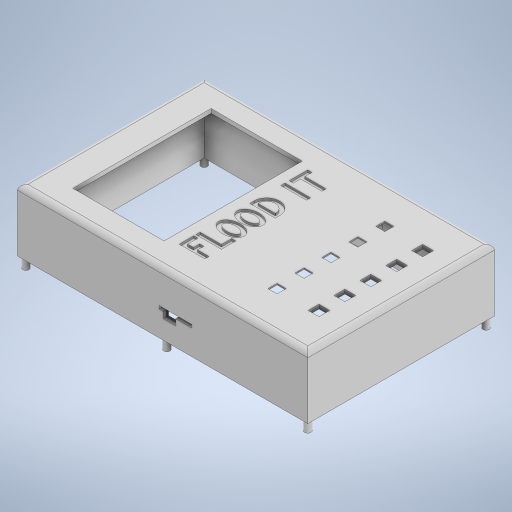
# Autodesk Inventor part: CaseTop3.0
Saved by Autodesk Inventor 2023 (Build 270158000, 158)
## iProperties
Created: 2022-11-29
Part Number: CaseTop3.0
Material: Generic
Document SubType Name: Modeling
Designer: spfow
Density: 1 g/cm^3
Appearance: Default
Author: spfow
Autodesk Inventor part; units mm, degrees
note: some values were not read from the file. Chosen so that the rebuilt part matches the saved one: offset side.
ref_plane "YZ Plane" through (0, 0, 0) normal (1, 0, 0) x (0, 1, 0)
ref_plane "XZ Plane" through (0, 0, 0) normal (0, 1, 0) x (-1, 0, 0)
ref_plane "XY Plane" through (0, 0, 0) normal (0, 0, 1) x (1, 0, 0)
sketch "Sketch1" plane through (0, 0, 0) normal (0, 1, 0) x (-1, 0, 0)
  line L0 (0, 0) -> (177.8, 0)
  line L1 (177.8, 0) -> (177.8, -114.3)
  line L2 (177.8, -114.3) -> (0, -114.3)
  line L3 (0, -114.3) -> (0, 0)
  dimension "d0" = 177.8
  dimension "d1" = 114.3
  constraints: 8 end point, 2 parallel, 1 horizontal, 1 perpendicular
  measures "d0" distance of L1.end L2.end
  measures "d1" distance of L0.end L1.end
extrude "Extrusion1" add sketch "Sketch1" along normal blind 38.1
sketch "Sketch2" plane through (0, 0, 0) normal (0, -1, 0) x (1, 0, 0)
  line L0 (-177.8, -114.3) -> (-177.8, 0) projected
  line L1 (0, 0) -> (-177.8, 0)
  line L2 (-177.8, 0) -> (-177.8, -114.3)
  line L3 (-177.8, -114.3) -> (0, -114.3)
  line L4 (0, -114.3) -> (0, 0)
  line L5 (-5.08, -5.08) -> (-172.72, -5.08)
  line L6 (-172.72, -5.08) -> (-172.72, -109.22)
  line L7 (-172.72, -109.22) -> (-5.08, -109.22)
  line L8 (-5.08, -109.22) -> (-5.08, -5.08)
  dimension "d4" = 5.08
  constraints: 16 end point, 4 parallel, 2 perpendicular, 1 horizontal, 3 other
  measures "d4" distance between parallel lines of L4 L8
extrude "Extrusion2" cut sketch "Sketch2" against normal blind 35.56 contours L8 L7 L6 L5
fillet "Fillet1" radius 3.175 4 edges at (-177.8, 38.1, -57.15) (-88.9, 38.1, 0) (-88.9, 38.1, -114.3) (0, 38.1, -57.15)
sketch "Sketch3" plane through (0, 38.1, 0) normal (0, 1, 0) x (1, 0, 0)
  line L0 (-177.8, 114.3) -> (-171.45, 114.3)
  line L1 (-171.45, 114.3) -> (-171.45, 0)
  line L2 (-171.45, 0) -> (-177.8, 0)
  line L3 (-177.8, 0) -> (-177.8, 114.3)
  line L4 (0, 114.3) -> (-177.8, 114.3) projected
  line L5 (-177.8, 114.3) -> (0, 114.3)
  line L6 (0, 114.3) -> (0, 107.95)
  line L7 (0, 107.95) -> (-177.8, 107.95)
  line L8 (-177.8, 107.95) -> (-177.8, 114.3)
  line L9 (-158.75, 99.5045) -> (-102.87, 99.5045)
  line L10 (-102.87, 99.5045) -> (-102.87, 14.7955)
  line L11 (-102.87, 14.7955) -> (-158.75, 14.7955)
  line L12 (-158.75, 14.7955) -> (-158.75, 99.5045)
  point P0 (0, 0)
  dimension "d8" = 6.35
  dimension "d9" = 6.35
  dimension "d10" = 55.88
  dimension "d11" = 84.709
  dimension "d12" = 14.7955
  dimension "d13" = 19.05
  constraints: 24 end point, 6 parallel, 3 horizontal, 3 perpendicular
  measures "d8" distance of L1.end L2.end
  measures "d9" distance of L5.end L6.end
  measures "d10" distance of L9.start L9.end
  measures "d11" distance of L9.end L10.end
  measures "d12" distance between parallel lines of L4 L9
  measures "d13" distance between parallel lines of L3 L12
extrude "Extrusion3" cut sketch "Sketch3" against normal blind 35.56 contours L9 L10 L11 L12
sketch "Sketch4" plane through (0, 38.1, 0) normal (0, 1, 0) x (1, 0, 0)
  line L0 (-96.52, 17.78) -> (-81.2088, 17.78)
  line L1 (-93.98, 20.32) -> (-93.98, 26.67)
  line L2 (-93.98, 26.67) -> (-96.52, 26.67)
  line L3 (-96.52, 26.67) -> (-96.52, 17.78)
  line L4 (-96.52, 17.78) -> (-80.899, 17.78)
  line L5 (-80.899, 17.78) -> (-80.899, 20.32)
  line L6 (-96.52, 23.1535) -> (-96.52, 17.78)
  line L7 (-87.884, 20.32) -> (-87.884, 24.13)
  line L8 (-87.884, 24.13) -> (-90.424, 24.13)
  line L9 (-90.424, 24.13) -> (-90.424, 20.32)
  line L10 (-80.899, 20.32) -> (-87.884, 20.32)
  line L11 (-90.424, 20.32) -> (-93.98, 20.32)
  line L12 (-102.87, 99.5045) -> (-102.87, 14.7955) projected
  line L13 (-177.8, 0) -> (0, 0) projected
  line L14 (-96.52, 27.94) -> (-80.899, 27.94)
  line L15 (-80.899, 27.94) -> (-80.899, 30.7699)
  line L16 (-83.439, 30.48) -> (-96.52, 30.48)
  line L17 (-96.52, 30.48) -> (-96.52, 27.94)
  line L18 (-83.0828, 27.94) -> (-80.899, 27.94)
  line L19 (-80.899, 27.94) -> (-80.899, 36.83)
  line L20 (-80.899, 36.83) -> (-83.439, 36.83)
  line L21 (-83.439, 36.83) -> (-83.439, 30.48)
  ellipse E0 centre (-88.7095, 41.91) end of major axis (-96.52, 41.91) minor radius 5.334
  ellipse E1 centre (-88.7095, 53.34) end of major axis (-96.52, 53.34) minor radius 5.334
  line L22 (-96.52, 60.96) -> (-80.899, 60.96)
  line L23 (-80.899, 60.96) -> (-80.899, 63.754)
  line L24 (-96.52, 63.754) -> (-96.52, 60.96)
  ellipse E2 centre (-88.7095, 63.754) end of major axis (-96.52, 63.754) minor radius 7.62 (-80.899, 63.754) -> (-96.52, 63.754) ccw
  line L25 (-93.98, 63.754) -> (-93.98, 63.5)
  line L26 (-93.98, 63.5) -> (-83.439, 63.5)
  line L27 (-83.439, 63.5) -> (-83.439, 63.754)
  line L28 (-96.52, 82.55) -> (-80.899, 82.55)
  line L29 (-80.899, 82.55) -> (-80.899, 80.01)
  line L30 (-80.899, 80.01) -> (-96.52, 80.01)
  line L31 (-96.52, 80.01) -> (-96.52, 82.55)
  line L32 (-93.98, 89.535) -> (-80.899, 89.535)
  line L33 (-80.899, 89.535) -> (-80.899, 92.075)
  line L34 (-80.899, 92.075) -> (-93.98, 92.075)
  line L35 (-96.52, 94.8241) -> (-96.52, 91.9305)
  line L36 (-96.52, 85.09) -> (-93.98, 85.09)
  line L37 (-93.98, 96.52) -> (-96.52, 96.52)
  line L38 (-96.52, 96.52) -> (-96.52, 85.09)
  line L39 (-93.98, 85.09) -> (-93.98, 89.535)
  line L40 (-93.98, 92.075) -> (-93.98, 96.52)
  spline S0 degree 5 poles (-93.98, 41.91) (-93.9809, 41.6813) (-93.9169, 41.4527) (-93.811, 41.2473) (-93.4267, 40.6846) (-92.8861, 40.2564) (-92.5045, 40.0177) (-91.5531, 39.5478) (-90.5271, 39.2718) (-89.9251, 39.1679) (-88.7095, 39.0641) (-87.4939, 39.1679) (-86.8919, 39.2718) (-85.866, 39.5478) (-84.9145, 40.0176) (-84.5332, 40.2563) (-83.9921, 40.6845) (-83.6083, 41.2473) (-83.5012, 41.4526) (-83.3764, 41.91) (-83.5012, 42.3674) (-83.6083, 42.5727) (-83.9921, 43.1355) (-84.5332, 43.5637) (-84.9145, 43.8024) (-85.866, 44.2722) (-86.8919, 44.5482) (-87.4939, 44.6521) (-88.7095, 44.7559) (-89.9251, 44.6521) (-90.5271, 44.5482) (-91.5531, 44.2722) (-92.5045, 43.8023) (-92.8861, 43.5636) (-93.4267, 43.1354) (-93.811, 42.5727) (-93.9169, 42.3673) (-93.9809, 42.1387) (-93.98, 41.91) knots 0 0 0 0 0 0 0.044471 0.044471 0.044471 0.131758 0.131758 0.131758 0.25 0.25 0.25 0.36824 0.36824 0.36824 0.455522 0.455522 0.455522 0.5 0.5 0.5 0.544478 0.544478 0.544478 0.63176 0.63176 0.63176 0.75 0.75 0.75 0.868242 0.868242 0.868242 0.955529 0.955529 0.955529 1 1 1 1 1 1
  spline S1 degree 5 poles (-93.98, 53.34) (-93.9809, 53.1113) (-93.9169, 52.8827) (-93.811, 52.6773) (-93.4267, 52.1146) (-92.8861, 51.6864) (-92.5045, 51.4477) (-91.5531, 50.9778) (-90.5271, 50.7018) (-89.9251, 50.5979) (-88.7095, 50.4941) (-87.4939, 50.5979) (-86.8919, 50.7018) (-85.866, 50.9778) (-84.9145, 51.4476) (-84.5332, 51.6863) (-83.9921, 52.1145) (-83.6083, 52.6773) (-83.5012, 52.8826) (-83.3764, 53.34) (-83.5012, 53.7974) (-83.6083, 54.0027) (-83.9921, 54.5655) (-84.5332, 54.9937) (-84.9145, 55.2324) (-85.866, 55.7022) (-86.8919, 55.9782) (-87.4939, 56.0821) (-88.7095, 56.1859) (-89.9251, 56.0821) (-90.5271, 55.9782) (-91.5531, 55.7022) (-92.5045, 55.2323) (-92.8861, 54.9936) (-93.4267, 54.5654) (-93.811, 54.0027) (-93.9169, 53.7973) (-93.9809, 53.5687) (-93.98, 53.34) knots 0 0 0 0 0 0 0.044471 0.044471 0.044471 0.131758 0.131758 0.131758 0.25 0.25 0.25 0.36824 0.36824 0.36824 0.455522 0.455522 0.455522 0.5 0.5 0.5 0.544478 0.544478 0.544478 0.63176 0.63176 0.63176 0.75 0.75 0.75 0.868242 0.868242 0.868242 0.955529 0.955529 0.955529 1 1 1 1 1 1
  spline S2 degree 5 poles (-83.439, 63.754) (-83.4391, 64.309) (-83.5178, 64.8639) (-83.675, 65.404) (-84.3507, 66.8995) (-85.581, 68.0474) (-86.5678, 68.5716) (-88.7095, 69.0964) (-90.8512, 68.5716) (-91.838, 68.0474) (-93.0683, 66.8995) (-93.744, 65.404) (-93.9012, 64.8639) (-93.9799, 64.309) (-93.98, 63.754) knots 0 0 0 0 0 0 0.170659 0.170659 0.170659 0.5 0.5 0.5 0.829341 0.829341 0.829341 1 1 1 1 1 1
  point P0 (-96.52, 93.3773)
  point P1 (-88.9, 0)
  point P2 (-95.25, 85.09)
  dimension "d32" = 5.334
  dimension "d33" = 7.8105
  dimension "d36" = 7.8105
  dimension "d37" = 5.334
  dimension "d42" = 7.62
  dimension "d43" = 2.54
  dimension "d16" = 2.54
  dimension "d17" = 3.556
  dimension "d18" = 2.54
  dimension "d19" = 6.985
  dimension "d20" = 8.89
  dimension "d21" = 6.35
  dimension "d22" = 3.81
  dimension "d23" = 3.81
  dimension "d24" = 6.35
  dimension "d25" = 17.78
  dimension "d26" = 2.54
  dimension "d27" = 2.54
  dimension "d28" = 6.35
  dimension "d29" = 15.621
  dimension "d30" = 6.35
  dimension "d31" = 27.94
  dimension "d34" = 14.1605
  dimension "d35" = 41.91
  dimension "d38" = 14.1605
  dimension "d39" = 53.34
  dimension "d40" = 2.54
  dimension "d41" = 2.54
  dimension "d44" = 6.35
  dimension "d45" = 15.621
  dimension "d46" = 60.96
  dimension "d47" = 2.794
  dimension "d48" = 63.754
  dimension "d49" = 14.1605
  dimension "d50" = 2.54
  dimension "d51" = 15.621
  dimension "d52" = 4.445
  dimension "d53" = 4.445
  dimension "d54" = 2.54
  dimension "d55" = 2.54
  dimension "d56" = 6.35
  dimension "d57" = 80.01
  dimension "d58" = 2.54
  dimension "d59" = 13.081
  dimension "d62" = 2.9845
  dimension "d63" = 2.9845
  constraints: 78 end point, 20 parallel, 10 perpendicular, 8 horizontal, 5 point on line, 3 midpoint, 13 other
  measures "d16" distance of L1.end L2.end
  measures "d17" distance of L9.end L1.start
  measures "d18" distance of L7.end L8.end
  measures "d19" distance of L5.end L7.start
  measures "d20" distance of L2.end L0.start
  measures "d21" distance of L1.start L1.end
  measures "d22" distance of L8.end L9.end
  measures "d23" distance of L7.start L7.end
  measures "d24" distance between parallel lines of L12 L3
  measures "d25" distance between parallel lines of L13 L0
  measures "d26" distance of L16.end L14.start
  measures "d27" distance of L19.end L20.end
  measures "d28" distance of L20.end L16.start
  measures "d29" distance of L14.start L14.end
  measures "d30" distance between parallel lines of L12 L17
  measures "d31" distance between parallel lines of L13 L14
  measures "d34" distance from line of L12 point (-88.71, 41.91)
  measures "d35" distance from line of L13 point (-88.71, 41.91)
  measures "d38" distance from line of L12 point (-88.71, 53.34)
  measures "d39" distance from line of L13 point (-88.71, 53.34)
  measures "d44" distance between parallel lines of L12 L24
  measures "d45" distance of L22.start L22.end
  measures "d46" distance between parallel lines of L13 L22
  measures "d47" distance of L24.start L22.start
  measures "d48" distance from line of L13 point (-88.71, 63.754)
  measures "d49" distance from line of L12 point (-88.71, 63.754)
  measures "d50" distance of L30.end L28.start
  measures "d51" distance of L29.end L30.end
  measures "d52" distance of L36.end L32.start
  measures "d53" distance of L34.end L37.start
  measures "d54" distance between parallel lines of L32 L34
  measures "d55" distance between parallel lines of L40 L38
  measures "d56" distance from line of L12 point (-96.52, 93.377)
  measures "d57" distance from line of point (-88.9, 0) L30
  measures "d58" distance from line of L28 point (-95.25, 85.09)
  measures "d59" distance of L32.start L32.end
  measures "d62" distance from line of L12.start L37
  measures "d63" distance from line of L12.end L0
extrude "Extrusion4" cut sketch "Sketch4" against normal blind 1.27
sketch "Sketch5" plane through (0, 38.1, 0) normal (0, 1, 0) x (1, 0, 0)
  line L0 (-45.72, 21.3678) -> (-40.1955, 21.3678)
  line L1 (-40.1955, 21.3678) -> (-40.1955, 26.8923)
  line L2 (-40.1955, 26.8923) -> (-45.72, 26.8923)
  line L3 (-45.72, 26.8923) -> (-45.72, 21.3678)
  line L4 (-45.72, 37.8778) -> (-40.1955, 37.8778)
  line L5 (-40.1955, 37.8778) -> (-40.1955, 43.4023)
  line L6 (-40.1955, 43.4023) -> (-45.72, 43.4023)
  line L7 (-45.72, 43.4023) -> (-45.72, 37.8778)
  line L8 (-45.72, 54.3877) -> (-40.1955, 54.3877)
  line L9 (-40.1955, 54.3877) -> (-40.1955, 59.9123)
  line L10 (-40.1955, 59.9123) -> (-45.72, 59.9123)
  line L11 (-45.72, 59.9123) -> (-45.72, 54.3877)
  line L12 (-45.72, 70.8978) -> (-40.1955, 70.8978)
  line L13 (-40.1955, 70.8978) -> (-40.1955, 76.4222)
  line L14 (-40.1955, 76.4222) -> (-45.72, 76.4222)
  line L15 (-45.72, 76.4222) -> (-45.72, 70.8978)
  line L16 (-45.72, 87.4077) -> (-40.1955, 87.4077)
  line L17 (-40.1955, 87.4077) -> (-40.1955, 92.9322)
  line L18 (-40.1955, 92.9322) -> (-45.72, 92.9322)
  line L19 (-45.72, 92.9322) -> (-45.72, 87.4077)
  line L20 (0, 114.3) -> (-177.8, 114.3) projected
  line L21 (-177.8, 0) -> (0, 0) projected
  line L22 (-102.87, 99.5045) -> (-102.87, 14.7955) projected
  point P0 (-45.72, 73.66)
  dimension "d64" = 5.5245
  dimension "d65" = 5.5245
  dimension "d66" = 5.5245
  dimension "d67" = 5.5245
  dimension "d68" = 5.5245
  dimension "d69" = 5.5245
  dimension "d70" = 16.51
  dimension "d71" = 16.51
  dimension "d72" = 16.51
  dimension "d73" = 16.51
  dimension "d74" = 21.3678
  dimension "d76" = 57.15
  dimension "d224" = 21.3678
  constraints: 40 end point, 10 parallel, 8 point on line, 5 horizontal, 5 perpendicular, 1 midpoint
  measures "d64" distance of L2.end L0.start
  measures "d65" distance of L6.end L4.start
  measures "d66" distance of L10.end L8.start
  measures "d67" distance of L14.end L12.start
  measures "d68" distance of L18.end L16.start
  measures "d69" distance of L17.end L18.end
  measures "d70" distance of L5.end L1.end
  measures "d71" distance of L9.end L5.end
  measures "d72" distance of L13.end L9.end
  measures "d73" distance of L17.end L13.end
  measures "d74" distance between parallel lines of L20 L18
  measures "d76" distance from line of point (-45.72, 73.66) L22
  measures "d224" distance between parallel lines of L21 L0
extrude "Extrusion5" cut sketch "Sketch5" against normal blind 25.4
sketch "Sketch6" plane through (0, 35.56, 0) normal (0, -1, 0) x (1, 0, 0)
  line L0 (-45.72, -87.4077) -> (-45.72, -92.9322) projected
  line L1 (-45.72, -92.9322) -> (-40.1955, -92.9322)
  line L2 (-40.1955, -92.9322) -> (-40.1955, -87.4077)
  line L3 (-40.1955, -87.4077) -> (-45.72, -87.4077)
  line L4 (-45.72, -87.4077) -> (-45.72, -92.9322)
  line L5 (-45.72, -76.4222) -> (-40.1955, -76.4222) projected
  line L6 (-45.72, -70.8978) -> (-40.1955, -70.8978) projected
  line L7 (-45.72, -76.4222) -> (-40.1955, -76.4222)
  line L8 (-40.1955, -76.4222) -> (-40.1955, -70.8978)
  line L9 (-40.1955, -70.8978) -> (-45.72, -70.8978)
  line L10 (-45.72, -70.8978) -> (-45.72, -76.4222)
  line L11 (-45.72, -54.3877) -> (-45.72, -59.9123) projected
  line L12 (-45.72, -54.3877) -> (-40.1955, -54.3877) projected
  line L13 (-45.72, -59.9123) -> (-40.1955, -59.9123)
  line L14 (-40.1955, -59.9123) -> (-40.1955, -54.3877)
  line L15 (-40.1955, -54.3877) -> (-45.72, -54.3877)
  line L16 (-45.72, -54.3877) -> (-45.72, -59.9123)
  line L17 (-45.72, -37.8778) -> (-45.72, -43.4023) projected
  line L18 (-40.1955, -37.8778) -> (-45.72, -37.8778) projected
  line L19 (-45.72, -43.4023) -> (-40.1955, -43.4023)
  line L20 (-40.1955, -43.4023) -> (-40.1955, -37.8778)
  line L21 (-40.1955, -37.8778) -> (-45.72, -37.8778)
  line L22 (-45.72, -37.8778) -> (-45.72, -43.4023)
  line L23 (-45.72, -21.3678) -> (-45.72, -26.8923) projected
  line L24 (-45.72, -26.8923) -> (-40.1955, -26.8923)
  line L25 (-40.1955, -26.8923) -> (-40.1955, -21.3678)
  line L26 (-40.1955, -21.3678) -> (-45.72, -21.3678)
  line L27 (-45.72, -21.3678) -> (-45.72, -26.8923)
  line L28 (-46.736, -86.3917) -> (-39.1795, -86.3917)
  line L29 (-39.1795, -86.3917) -> (-39.1795, -93.9483)
  line L30 (-39.1795, -93.9483) -> (-46.736, -93.9483)
  line L31 (-46.736, -93.9483) -> (-46.736, -86.3917)
  line L32 (-46.736, -77.4383) -> (-39.1795, -77.4383)
  line L33 (-39.1795, -77.4383) -> (-39.1795, -69.8817)
  line L34 (-39.1795, -69.8817) -> (-46.736, -69.8817)
  line L35 (-46.736, -69.8817) -> (-46.736, -77.4383)
  line L36 (-39.1795, -60.9282) -> (-46.736, -60.9282)
  line L37 (-46.736, -60.9282) -> (-46.736, -53.3718)
  line L38 (-46.736, -53.3718) -> (-39.1795, -53.3718)
  line L39 (-39.1795, -53.3718) -> (-39.1795, -60.9282)
  line L40 (-39.1795, -44.4182) -> (-46.736, -44.4182)
  line L41 (-46.736, -44.4182) -> (-46.736, -36.8618)
  line L42 (-46.736, -36.8618) -> (-39.1795, -36.8618)
  line L43 (-39.1795, -36.8618) -> (-39.1795, -44.4182)
  line L44 (-39.1795, -27.9082) -> (-46.736, -27.9082)
  line L45 (-46.736, -27.9082) -> (-46.736, -20.3518)
  line L46 (-46.736, -20.3518) -> (-39.1795, -20.3518)
  line L47 (-39.1795, -20.3518) -> (-39.1795, -27.9082)
  line L48 (-49.1173, -100.3999) -> (-36.7983, -100.3999)
  line L49 (-36.7983, -100.3999) -> (-36.7983, -15.9449)
  line L50 (-36.7983, -15.9449) -> (-49.1173, -15.9449)
  line L51 (-49.1173, -15.9449) -> (-49.1173, -100.3999)
  line L52 (-21.844, -22.098) -> (-15.24, -22.098)
  line L53 (-15.24, -22.098) -> (-15.24, -28.702)
  line L54 (-15.24, -28.702) -> (-21.844, -28.702)
  line L55 (-21.844, -28.702) -> (-21.844, -22.098)
  line L56 (-21.844, -44.577) -> (-21.844, -37.973)
  line L57 (-15.24, -37.973) -> (-15.24, -44.577)
  line L58 (-15.24, -44.577) -> (-21.844, -44.577)
  line L59 (-21.844, -37.973) -> (-15.24, -37.973)
  line L60 (-21.844, -60.452) -> (-21.844, -53.848)
  line L61 (-15.24, -53.848) -> (-15.24, -60.452)
  line L62 (-15.24, -60.452) -> (-21.844, -60.452)
  line L63 (-21.844, -53.848) -> (-15.24, -53.848)
  line L64 (-21.844, -76.327) -> (-21.844, -69.723)
  line L65 (-15.24, -69.723) -> (-15.24, -76.327)
  line L66 (-15.24, -76.327) -> (-21.844, -76.327)
  line L67 (-21.844, -69.723) -> (-15.24, -69.723)
  line L68 (-21.844, -92.202) -> (-21.844, -85.598)
  line L69 (-15.24, -85.598) -> (-15.24, -92.202)
  line L70 (-15.24, -92.202) -> (-21.844, -92.202)
  line L71 (-21.844, -85.598) -> (-15.24, -85.598)
  line L72 (-172.72, -5.08) -> (-5.08, -5.08) projected
  line L73 (-5.08, -109.22) -> (-172.72, -109.22) projected
  line L74 (-5.08, -5.08) -> (-5.08, -109.22) projected
  point P0 (0, 0)
  point P1 (-42.9578, -93.9483)
  point P2 (-42.9578, -100.3999)
  point P3 (-42.9578, -15.9449)
  point P4 (-42.9578, -20.3518)
  dimension "d189" = 1.016
  dimension "d190" = 1.016
  dimension "d191" = 1.016
  dimension "d192" = 1.016
  dimension "d193" = 1.016
  dimension "d194" = 12.319
  dimension "d195" = 2.3813
  dimension "d197" = 84.455
  dimension "d198" = 6.4516
  dimension "d199" = 4.4069
  dimension "d248" = 6.604
  dimension "d249" = 6.604
  dimension "d252" = 15.875
  dimension "d257" = 17.018
  dimension "d258" = 17.018
  dimension "d259" = 10.16
  constraints: 128 end point, 24 parallel, 12 perpendicular, 7 horizontal, 4 midpoint, 1 collinear, 1 vertical, 46 other
  measures "d189" distance between parallel lines of L3 L28
  measures "d190" distance between parallel lines of L10 L35
  measures "d191" distance between parallel lines of L13 L36
  measures "d192" distance between parallel lines of L19 L40
  measures "d193" distance between parallel lines of L24 L44
  measures "d194" distance of L49.end L50.end
  measures "d195" distance between parallel lines of L31 L51
  measures "d197" distance of L50.end L48.start
  measures "d198" distance of point (-42.958, -93.948) point (-42.958, -100.4)
  measures "d199" distance of point (-42.958, -15.945) point (-42.958, -20.352)
  measures "d248" distance of L53.end L54.end
  measures "d249" distance of L52.end L53.end
  measures "d252" distance of L54.end L56.start
  measures "d257" distance between parallel lines of L72 L52
  measures "d258" distance between parallel lines of L73 L70
  measures "d259" distance between parallel lines of L74 L53
extrude "Extrusion9" cut sketch "Sketch6" against normal blind 1.7463 contours L28 L29 L30 L31 | L35 L34 L33 L32 | L36 L37 L38 L39 | L40 L41 L42 L43 | L44 L45 L46 L47
sketch "Sketch8" plane through (0, 35.56, 0) normal (0, -1, 0) x (1, 0, 0)
  line L0 (-102.87, -14.7955) -> (-102.87, -99.5045) projected
  line L1 (-102.87, -14.7955) -> (-160.9725, -14.7955)
  line L2 (-160.9725, -14.7955) -> (-160.9725, -8.4455)
  line L3 (-160.9725, -8.4455) -> (-102.87, -8.4455)
  line L4 (-102.87, -8.4455) -> (-102.87, -14.7955)
  line L5 (-158.75, -99.5045) -> (-102.87, -99.5045) projected
  line L6 (-102.87, -99.5045) -> (-160.9725, -99.5045)
  line L7 (-160.9725, -99.5045) -> (-160.9725, -106.4895)
  line L8 (-160.9725, -106.4895) -> (-102.87, -106.4895)
  line L9 (-102.87, -106.4895) -> (-102.87, -99.5045)
  line L10 (-102.87, -8.4455) -> (-96.52, -8.4455)
  line L11 (-96.52, -8.4455) -> (-96.52, -14.7955)
  line L12 (-96.52, -14.7955) -> (-102.87, -14.7955)
  line L13 (-102.87, -14.7955) -> (-102.87, -8.4455)
  line L14 (-102.87, -99.5045) -> (-96.52, -99.5045)
  line L15 (-96.52, -99.5045) -> (-96.52, -106.4895)
  line L16 (-96.52, -106.4895) -> (-102.87, -106.4895)
  line L17 (-102.87, -106.4895) -> (-102.87, -99.5045)
  line L18 (-160.9725, -99.5045) -> (-167.3225, -99.5045)
  line L19 (-167.3225, -99.5045) -> (-167.3225, -106.4895)
  line L20 (-167.3225, -106.4895) -> (-160.9725, -106.4895)
  line L21 (-160.9725, -106.4895) -> (-160.9725, -99.5045)
  line L22 (-160.9725, -8.4455) -> (-167.3225, -8.4455)
  line L23 (-167.3225, -8.4455) -> (-167.3225, -12.827)
  line L24 (-167.3225, -12.827) -> (-160.9725, -12.827)
  line L25 (-160.9725, -12.827) -> (-160.9725, -8.4455)
  line L26 (-104.6278, -10.033) -> (-157.9678, -10.033)
  line L27 (-157.9678, -10.033) -> (-157.9678, -15.113)
  line L28 (-157.9678, -15.113) -> (-104.6278, -15.113)
  line L29 (-104.6278, -15.113) -> (-104.6278, -10.033)
  point P0 (0, 0)
  dimension "d126" = 6.35
  dimension "d127" = 6.985
  dimension "d128" = 6.35
  dimension "d129" = 6.35
  dimension "d130" = 6.35
  dimension "d131" = 53.34
  dimension "d132" = 5.08
  dimension "d245" = 1.5875
  constraints: 56 end point, 14 parallel, 7 horizontal, 7 perpendicular, 2 point on line
  measures "d126" distance of L3.end L0.start
  measures "d127" distance of L8.end L0.end
  measures "d128" distance of L11.end L12.end
  measures "d129" distance of L20.end L19.end
  measures "d130" distance of L24.end L23.end
  measures "d131" distance of L28.end L27.end
  measures "d132" distance between parallel lines of L28 L26
  measures "d245" distance between parallel lines of L3 L26
extrude "Extrusion10" cut sketch "Sketch8" against normal blind 1.27 contours L29 L28 L27 L1 | L1 L27 L26 L29
extrude "Extrusion11" cut sketch "Sketch6" against normal blind 0.9525 contours L51 L50 L49 L48
sketch "Sketch9" plane through (-177.8, 0, 0) normal (0, 0, 1) x (1, 0, 0)
  line L0 (74.93, 35.56) -> (19.05, 35.56) projected
  line L1 (172.72, 0) -> (5.08, 0) projected
  line L2 (74.93, 35.56) -> (125.73, 35.56)
  line L3 (125.73, 35.56) -> (125.73, 0)
  line L4 (125.73, 0) -> (74.93, 0)
  line L5 (74.93, 0) -> (74.93, 35.56)
  line L6 (86.741, 17.145) -> (106.68, 17.145)
  line L7 (106.68, 17.145) -> (106.68, 15.3035)
  line L8 (106.68, 15.3035) -> (86.741, 15.3035)
  line L9 (86.741, 15.3035) -> (86.741, 17.145)
  line L10 (89.281, 15.3035) -> (96.901, 15.3035)
  line L11 (96.901, 15.3035) -> (96.901, 11.4935)
  line L12 (96.901, 11.4935) -> (89.281, 11.4935)
  line L13 (89.281, 11.4935) -> (89.281, 15.3035)
  line L14 (0, 34.925) -> (177.8, 34.925) projected
  line L15 (0, 0) -> (0, 34.925) projected
  line L16 (177.8, 0) -> (177.8, 34.925) projected
  dimension "d144" = 50.8
  dimension "d145" = 19.939
  dimension "d146" = 1.8415
  dimension "d147" = 7.62
  dimension "d148" = 3.81
  dimension "d149" = 2.54
  dimension "d150" = 17.78
  dimension "d187" = 71.12
  constraints: 24 end point, 6 parallel, 3 horizontal, 3 perpendicular, 2 point on line
  measures "d144" distance of L3.end L4.end
  measures "d145" distance of L6.start L6.end
  measures "d146" distance of L6.end L7.end
  measures "d147" distance of L11.end L12.end
  measures "d148" distance of L10.end L11.end
  measures "d149" distance between parallel lines of L9 L13
  measures "d150" distance between parallel lines of L14 L6
  measures "d187" distance between parallel lines of L16 L7
extrude "Extrusion12" cut sketch "Sketch9" against normal blind 5.08 contours L6 L7 L8 L9 | L8 L11 L12 L13
sketch "Sketch10" plane through (-5.08, 0, -5.08) normal (0, 0, -1) x (-1, 0, 0)
  line L0 (83.439, 11.4935) -> (75.819, 11.4935) projected
  line L1 (83.439, 15.3035) -> (85.979, 15.3035) projected
  line L2 (75.819, 11.4935) -> (83.439, 11.4935)
  line L3 (83.439, 11.4935) -> (83.439, 15.3035)
  line L4 (75.819, 15.3035) -> (75.819, 11.4935)
  line L5 (75.819, 15.3035) -> (66.04, 15.3035) projected
  line L6 (85.979, 17.145) -> (85.979, 15.3035) projected
  line L7 (85.979, 15.3035) -> (85.979, 17.145)
  line L8 (85.979, 17.145) -> (66.04, 17.145)
  line L9 (66.04, 17.145) -> (66.04, 15.3035)
  line L10 (66.04, 15.3035) -> (75.819, 15.3035)
  line L11 (83.439, 15.3035) -> (85.979, 15.3035)
  line L12 (73.914, 9.5885) -> (85.344, 9.5885)
  line L13 (85.344, 9.5885) -> (85.344, 13.3985)
  line L14 (85.344, 13.3985) -> (87.884, 13.3985)
  line L15 (87.884, 13.3985) -> (87.884, 19.05)
  line L16 (87.884, 19.05) -> (64.135, 19.05)
  line L17 (64.135, 19.05) -> (64.135, 13.3985)
  line L18 (64.135, 13.3985) -> (73.914, 13.3985)
  line L19 (73.914, 13.3985) -> (73.914, 9.5885)
  line L20 (73.914, 13.3985) -> (73.914, 15.3035)
  line L21 (85.344, 13.3985) -> (85.344, 15.3035)
  point P0 (-5.08, 0)
  dimension "d153" = 1.905
  constraints: 36 end point, 9 parallel, 7 perpendicular, 3 horizontal, 2 point on line, 7 other
  measures "d153" distance between parallel lines of L4 L19
extrude "Extrusion13" cut sketch "Sketch10" against normal blind 3.175 contours L3 L1 L21 L13 L12 L19 L20 L5 L4 L0 | L1 L6 L8 L9 L5 L20 L18 L17 L16 L15 L14 L21
sketch "Sketch11" plane through (0, 0, -114.3) normal (0, 0, -1) x (-1, 0, 0)
  line L0 (63.5, 23.495) -> (75.946, 23.495)
  line L1 (75.946, 23.495) -> (75.946, 16.256)
  line L2 (75.946, 16.256) -> (63.5, 16.256)
  line L3 (63.5, 16.256) -> (63.5, 23.495)
  line L4 (0, 0) -> (0, 34.925) projected
  circle A0 centre (69.723, 19.8755) radius 3.6195
  line L5 (0, 34.925) -> (177.8, 34.925) projected
  dimension "d156" = 7.239
  dimension "d157" = 63.5
  dimension "d158" = 12.446
  dimension "d164" = 11.43
  dimension "d219" = 7.239
  dimension "d220" = 3.6195
  dimension "d221" = 6.223
  constraints: 8 end point, 2 parallel, 1 centre point, 1 horizontal, 1 perpendicular
  measures "d156" distance of L0.end L1.end
  measures "d157" distance between parallel lines of L4 L3
  measures "d158" distance of L0.start L0.end
  measures "d164" distance between parallel lines of L5 L0
  measures "d219" diameter of A0
  measures "d220" distance from line of L0 A0.centre
  measures "d221" distance from line of L3 A0.centre
extrude "Extrusion14" cut sketch "Sketch11" against normal blind 6.35 contours A0
sketch "Sketch12" plane through (-172.72, 0, -109.22) normal (0, 0, 1) x (1, 0, 0)
  line L0 (96.774, 16.256) -> (109.22, 16.256)
  line L1 (109.22, 16.256) -> (109.22, 23.495)
  line L2 (109.22, 23.495) -> (96.774, 23.495)
  line L3 (96.774, 23.495) -> (96.774, 16.256)
  circle A0 centre (102.997, 19.8755) radius 3.6195 projected
  line L4 (96.774, 16.256) -> (109.22, 23.495) construction
  line L5 (109.22, 16.256) -> (96.774, 23.495) construction
  point P0 (172.72, 0)
  point P1 (102.997, 16.256)
  point P2 (102.997, 23.495)
  dimension "d161" = 12.446
  dimension "d222" = 7.239
  constraints: 12 end point, 2 midpoint, 2 parallel, 1 horizontal, 1 perpendicular
  measures "d161" distance of L0.start L0.end
  measures "d222" distance between parallel lines of L0 L2
extrude "Extrusion15" cut sketch "Sketch12" against normal blind 2.0574 contours L3 L2 A0 L0 | A0 L2 L1 L0
sketch "Sketch16" plane through (0, 0, 0) normal (0, -1, 0) x (1, 0, 0)
  circle A0 centre (-2.54, -2.54) radius 1.905
  circle A1 centre (-2.54, -111.76) radius 1.905
  circle A2 centre (-88.9, -111.76) radius 1.905
  circle A3 centre (-88.9, -2.54) radius 1.905
  circle A4 centre (-175.26, -2.54) radius 1.905
  circle A5 centre (-175.26, -111.76) radius 1.905
  line L0 (0, 0) -> (0, -114.3) projected
  line L1 (-177.8, 0) -> (0, 0) projected
  line L2 (0, -114.3) -> (-177.8, -114.3) projected
  line L3 (-177.8, -114.3) -> (-177.8, 0) projected
  line L4 (-172.72, -5.08) -> (-5.08, -5.08) projected
  dimension "d225" = 3.81
  dimension "d226" = 3.81
  dimension "d227" = 3.81
  dimension "d228" = 3.81
  dimension "d229" = 3.81
  dimension "d230" = 3.81
  dimension "d231" = 2.54
  dimension "d232" = 2.54
  dimension "d233" = 2.54
  dimension "d234" = 2.54
  dimension "d235" = 2.54
  dimension "d236" = 2.54
  dimension "d237" = 2.54
  dimension "d238" = 2.54
  dimension "d239" = 2.54
  dimension "d240" = 2.54
  dimension "d241" = 88.9
  dimension "d242" = 88.9
  constraints: 6 centre point
  measures "d225" diameter of A0
  measures "d226" diameter of A1
  measures "d227" diameter of A2
  measures "d228" diameter of A3
  measures "d229" diameter of A4
  measures "d230" diameter of A5
  measures "d231" distance from line of L0 A0.centre
  measures "d232" distance from line of L1 A0.centre
  measures "d233" distance from line of L0 A1.centre
  measures "d234" distance from line of L2 A1.centre
  measures "d235" distance from line of L2 A2.centre
  measures "d236" distance from line of L1 A3.centre
  measures "d237" distance from line of L3 A4.centre
  measures "d238" distance from line of L4 A4.centre
  measures "d239" distance from line of L2 A5.centre
  measures "d240" distance from line of L3 A5.centre
  measures "d241" distance from line of L0 A2.centre
  measures "d242" distance from line of L0 A3.centre
extrude "Extrusion19" add sketch "Sketch16" along normal blind 6.223 contours A0 | A1 | A2 | A3 | A4 | A5
extrude "Extrusion21" cut sketch "Sketch6" against normal blind 25.4 contours L52 L53 L54 L55 | L56 L59 L57 L58 | L60 L63 L61 L62 | L64 L67 L65 L66 | L68 L71 L69 L70
body "Solid1"
